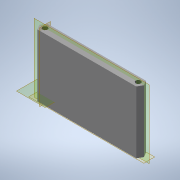
# Autodesk Inventor part: Steunstuk lang
Saved by Autodesk Inventor 2021 (Build 250183000, 183)
## iProperties
Created: 2021-02-03
Part Number: Steunstuk lang
Material: S235
Catalog Web Link: http://emmausbovenbouw.op-weg.be/
Vendor: Emmaüsinstituut Bovenbouw Aalter
Document SubType Name: Modeling
Designer: Antho
Engineer: Declercq St.
Manufacturer: Standard
Standards Organization: Custom
Density: 7.86 g/cm^3
Appearance: Steel
Manager: PJ / DCS
Company: Emmaüs Bovenbouw Aalter
Title: Algemene titel
Subject: Specifieke titel
Author: Antho
Keywords: Ruwe Ø xxxxx
Comments: Opmerking
Autodesk Inventor part; units mm, degrees
sketch "Sketch2" plane through (0, 0, 0) normal (0, 0, 1) x (1, 0, 0)
  line L0 (0, 2.8582) -> (0, -2.8582) construction
  line L1 (-5.7775, 0) -> (5.7775, 0) construction
  line L2 (0, 0) -> (4, 0)
  line L3 (4, 0) -> (-4, 0)
  circle A0 centre (0, 0) radius 4
  line L4 (0, 0) -> (-2, 3.4641)
  line L5 (0, 0) -> (4, 0) construction
  line L6 (0, 0) -> (2, 3.4641)
  line L7 (0, 0) -> (4, 0) construction
  line L8 (0, 0) -> (4, 0)
  line L9 (0, 0) -> (2, -3.4641)
  line L10 (0, 0) -> (-2, -3.4641)
  line L11 (-2, 3.4641) -> (2, 3.4641)
  line L12 (2, 3.4641) -> (4, 0)
  line L13 (4, 0) -> (2, -3.4641)
  line L14 (2, -3.4641) -> (-2, -3.4641)
  line L15 (-2, -3.4641) -> (-4, 0)
  line L16 (-4, 0) -> (-2, 3.4641)
  dimension "d3" = 4
  dimension "d2" = 8
  dimension "d1" = 120
  dimension "d0" = 60
  constraints: 34 end point, 5 point on circle, 4 equal length, 3 coincident, 3 horizontal, 3 point on line, 2 midpoint, 1 centre point, 1 vertical
  measures "d3" distance of L2.start L2.end
  measures "d2" distance of L2.end L3.end
  measures "d1" angle of L5 L4
  measures "d0" angle of L7 L6
extrude "Extrusion1" add sketch "Sketch2" along normal blind 43.5 contours L6 L12 L2 | L10 L15 L3 | L3 L16 L4 | L4 L11 L6 | L2 L13 L9 | L9 L14 L10
sketch "Sketch3" plane through (0, 0, 43.5) normal (0, 0, 1) x (1, 0, 0)
  point P0 (0, 0)
  point P1 (0, 0)
  constraints: 1 coincident
hole "Hole1" at (0, 0, 43.5) direction (0, 0, -1) diameter 3.4587 depth 8 thread size "M4x0.5" class "6H" standard "ISO Metric profile"
sketch "Sketch4" plane through (0, 0, 0) normal (0, 0, -1) x (-1, 0, 0)
  point P0 (0, 0)
  point P1 (0, 0)
  constraints: 1 coincident
hole "Hole2" at (0, 0, 0) direction (0, 0, 1) diameter 3.4587 depth 10.8 thread size "M4x0.5" class "6H" standard "ISO Metric profile"
ref_plane "Work Plane1" through (0, 0, 5.4) normal (0, 0, -1) x (-1, 0, 0)
sketch "Sketch5" plane through (0, 0, 43.5) normal (0, 0, 1) x (1, 0, 0)
  line L0 (0, 0) -> (65.19, 0)
  line L1 (65.19, 0) -> (69.19, 0)
  line L2 (65.19, 0) -> (65.19, 3.464)
  line L3 (65.19, 3.464) -> (67.19, 3.464)
  line L4 (67.19, 3.464) -> (69.19, 0)
  line L5 (65.19, 3.464) -> (63.19, 3.464)
  line L6 (65.19, 0) -> (61.19, 0)
  line L7 (61.19, 0) -> (63.19, 3.464)
  line L8 (65.19, 0) -> (65.19, -3.464)
  line L9 (65.19, -3.464) -> (67.19, -3.464)
  line L10 (67.19, -3.464) -> (69.19, 0)
  line L11 (65.19, -3.464) -> (63.19, -3.464)
  line L12 (63.19, -3.464) -> (61.19, 0)
  line L13 (2, 3.4641) -> (-2, 3.4641) projected
  line L14 (0, 3.4641) -> (65.19, 3.464)
  line L15 (65.19, -3.464) -> (0, -3.4641)
  line L16 (-2, -3.4641) -> (2, -3.4641) projected
  line L17 (4, 0) -> (2, 3.4641) projected
  line L18 (0, 3.4641) -> (4, 0)
  line L19 (4, 0) -> (0, -3.4641)
  point P0 (2, 3.4641)
  dimension "d21" = 65.19
  dimension "d22" = 4
  dimension "d23" = 3.464
  dimension "d24" = 2
  dimension "d25" = 2
  dimension "d26" = 4
  dimension "d27" = 3.464
  dimension "d28" = 2
  dimension "d29" = 2
  constraints: 34 end point, 3 point on line, 2 horizontal, 2 midpoint, 2 perpendicular, 1 parallel, 1 vertical
  measures "d21" distance of L0.start L0.end
  measures "d22" distance of L0.end L1.end
  measures "d23" distance of L0.end L2.end
  measures "d24" distance of L2.end L3.end
  measures "d25" distance of L2.end L5.end
  measures "d26" distance of L0.end L6.end
  measures "d27" distance of L0.end L8.end
  measures "d28" distance of L8.end L9.end
  measures "d29" distance of L8.end L11.end
extrude "Extrusion2" add sketch "Sketch5" against normal blind 43.5 contours L17 L14 L7 L0 | L0 L12 L15 L19 | L7 L5 L2 L0 | L0 L8 L11 L12 | L2 L3 L4 L1 | L1 L10 L9 L8
sketch "Sketch6" plane through (0, 0, 43.5) normal (0, 0, 1) x (1, 0, 0)
  line L0 (0, 0) -> (65.19, 0)
  dimension "d32" = 65.19
  constraints: 2 end point, 1 coincident, 1 horizontal
  measures "d32" distance of L0.start L0.end
hole "Hole3" at (65.19, 0, 43.5) direction (0, 0, -1) diameter 3.4587 depth 8 thread size "M4x0.5" class "6H" standard "ISO Metric profile"
sketch "Sketch7" plane through (0, 0, 0) normal (0, 0, -1) x (-1, 0, 0)
  line L0 (0, 0) -> (-65.19, 0)
  dimension "d40" = 65.19
  constraints: 2 end point, 1 coincident, 1 horizontal
  measures "d40" distance of L0.start L0.end
hole "Hole4" at (65.19, 0, 0) direction (0, 0, 1) diameter 3.4587 depth 8 thread size "M4x0.5" class "6H" standard "ISO Metric profile"
body "Solid1"
